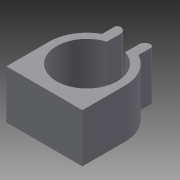
# Autodesk Inventor part: WireClip10
Saved by Autodesk Inventor 2015 SP1 (Build 190203100, 203)
## iProperties
Created: 2015-04-12
Part Number: WireClip10
Material: Generic
Document SubType Name: Modeling
Designer: Jack
Density: 1 g/cm^3
Appearance: Default
Author: Jack
Autodesk Inventor part; units mm, degrees
ref_plane "YZ Plane" through (0, 0, 0) normal (1, 0, 0) x (0, 1, 0)
ref_plane "XZ Plane" through (0, 0, 0) normal (0, 1, 0) x (-1, 0, 0)
ref_plane "XY Plane" through (0, 0, 0) normal (0, 0, 1) x (1, 0, 0)
sketch "Sketch3" plane through (0, 0, 0) normal (0, 0, 1) x (1, 0, 0)
  line L0 (-6.25, 1) -> (-6.25, 8)
  line L1 (6.25, 1) -> (6.25, 8)
  arc A0 (-1.5, 12.7697) -> (1.5, 12.7697) centre (0, 8) ccw
  line L2 (-3, 13.4829) -> (-3, 16)
  line L3 (-3, 16) -> (-1.5, 16)
  line L4 (1.5, 16) -> (3, 16)
  line L5 (3, 16) -> (3, 13.4829)
  arc A1 (-3, 13.4829) -> (-6.25, 8) centre (0, 8) ccw
  arc A2 (6.25, 8) -> (3, 13.4829) centre (0, 8) ccw
  line L6 (6.25, 1) -> (-6.25, 1)
  line L7 (-1.5, 16) -> (-1.5, 12.7697)
  line L8 (1.5, 12.7697) -> (1.5, 16)
  point P0 (0, 0)
  dimension "d10" = 10
  dimension "d12" = 8
  dimension "d13" = 1.5
  dimension "d21" = 1.25
  dimension "d22" = 1.25
  dimension "d24" = 7
  dimension "d25" = 8
  dimension "d26" = 3
  constraints: 18 end point, 6 point on circle, 3 centre point, 3 vertical, 2 equal length, 2 horizontal, 2 perpendicular, 2 point on line, 2 tangent, 1 coincident, 1 horizontal alignment, 1 vertical alignment
  measures "d10" diameter of A0
  measures "d12" distance from line of A1.centre L4
  measures "d13" distance of L4.start L4.end
  measures "d21" radial gap between concentric circles of A2 A0
  measures "d22" radial gap between concentric circles of A1 A0
  measures "d24" distance from line of A1.centre L6
  measures "d25" distance of point (0, 0) A1.centre
  measures "d26" distance between parallel lines of L8 L7
extrude "Extrusion1" add sketch "Sketch3" along normal blind 8
fillet "Fillet1" radius 1 2 edges at (-1.5, 16, 4) (1.5, 16, 4)
fillet "Fillet2" radius 0.5 2 edges at (3, 16, 4) (-3, 16, 4)
body "Solid1"
